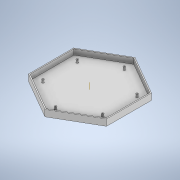
# Autodesk Inventor part: hexlight-top-led-nodule
Saved by Autodesk Inventor 2020 (Build 240168000, 168)
## iProperties
Created: 2019-09-27
Part Number: hexlight-top-led-nodule
Material: Generic
Document SubType Name: Modeling
Designer: Adam
Density: 1 g/cm^3
Appearance: Default
Author: Adam
Autodesk Inventor part; units mm, degrees
ref_plane "YZ Plane" through (0, 0, 0) normal (1, 0, 0) x (0, 1, 0)
ref_plane "XZ Plane" through (0, 0, 0) normal (0, 1, 0) x (-1, 0, 0)
ref_plane "XY Plane" through (0, 0, 0) normal (0, 0, 1) x (1, 0, 0)
sketch "Sketch1" plane through (0, 0, 0) normal (0, 1, 0) x (-1, 0, 0)
  line L0 (0, 85) -> (73.6122, 42.5)
  line L1 (73.6122, 42.5) -> (73.6122, -42.5)
  line L2 (73.6122, -42.5) -> (0, -85)
  line L3 (0, -85) -> (-73.6122, -42.5)
  line L4 (-73.6122, -42.5) -> (-73.6122, 42.5)
  line L5 (-73.6122, 42.5) -> (0, 85)
  point P0 (0, 0)
  point P1 (0, 0)
  dimension "d0" = 0
  dimension "d1" = 85
  constraints: 12 end point, 1 coincident, 13 other
  measures "d0" horizontal distance of point (0, 0) L0.start
  measures "d1" distance of L0.end L1.end
extrude "Extrusion1" add sketch "Sketch1" along normal blind 12
sketch "Sketch2" plane through (0, 12, 0) normal (0, 1, 0) x (1, 0, 0)
  line L0 (0, -82.6906) -> (-71.6122, -41.3453)
  line L1 (-71.6122, -41.3453) -> (-71.6122, 41.3453)
  line L2 (-71.6122, 41.3453) -> (0, 82.6906)
  line L3 (0, 82.6906) -> (71.6122, 41.3453)
  line L4 (71.6122, 41.3453) -> (71.6122, -41.3453)
  line L5 (71.6122, -41.3453) -> (0, -82.6906)
  line L6 (-73.6122, 42.5) -> (-73.6122, -42.5) projected
  point P0 (0, 0)
  point P1 (0, 0)
  point P2 (0, 0)
  dimension "d6" = 0
  dimension "d7" = 2
  constraints: 12 end point, 2 coincident, 13 other
  measures "d6" horizontal distance of point (0, 0) L0.start
  measures "d7" distance from line of L6 L0.end
extrude "Extrusion2" cut sketch "Sketch2" against normal blind 10
sketch "Sketch3" plane through (0, 2, 0) normal (0, 1, 0) x (1, 0, 0)
  circle A0 centre (0, -65) radius 2
  point P0 (0, 0)
  dimension "d10" = 4
  dimension "d11" = 65
  constraints: 1 centre point
  measures "d10" diameter of A0
  measures "d11" distance of point (0, 0) A0.centre
extrude "Extrusion3" add sketch "Sketch3" along normal blind 5
sketch "Sketch4" plane through (0, 7, 65) normal (0, 1, 0) x (1, 0, 0)
  point P0 (0, 65)
  point P1 (0, 0)
  point P2 (0, 0)
  dimension "d14" = 65
  dimension "d15" = 0
  measures "d14" distance of point (0, 65) point (0, 0)
  measures "d15" horizontal distance of point (0, 65) point (0, 0)
hole "Hole1" at (0, 7, 65) direction (0, -1, 0) diameter 1.5 end through all
pattern_circular "Circular Pattern1" count 6 over 360 about axis through (0, -10, 0) along (0, 1, 0) of "Extrusion3", "Hole1"
body "Solid1"
